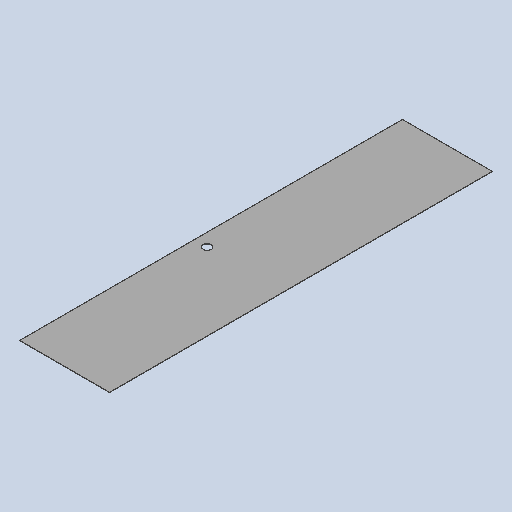
# Autodesk Inventor part: BSH 051 sheet in
Saved by Autodesk Inventor 2025 (Build 290162010, 162A)
## iProperties
Created: 2024-07-23
Part Number: BSH 051 sheet in
Material: 09g2s
Document SubType Name: Sheet Metal
Designer: admin
Mass: 40581.4 g
Surface Area: 34651.2 cm^2
Volume: 5169.6 cm^3
Density: 7.85 g/cm^3
Flat Pattern Width: 70 cm
Flat Pattern Length: 298 cm
Flat Pattern Area: 20860 cm^2
Sheet Metal Rule: AISI304 3mm Die 32
Sheet Metal Width: 700,000 mm
Sheet Metal Length: 2980,000 mm
Sheet Metal Area: 2086000,000 mm^2
Appearance: Default
Stock Number: БШК 051 лист внутренний
Author: admin
Autodesk Inventor part; units mm, degrees
ref_plane "YZ Plane" through (0, 0, 0) normal (1, 0, 0) x (0, 1, 0)
ref_plane "XZ Plane" through (0, 0, 0) normal (0, 1, 0) x (-1, 0, 0)
ref_plane "XY Plane" through (0, 0, 0) normal (0, 0, 1) x (1, 0, 0)
sketch "Sketch1" plane through (0, 0, 0) normal (0, 0, 1) x (1, 0, 0)
  line L0 (0, -1490) -> (700, -1490)
  line L1 (700, -1490) -> (700, 1490)
  line L2 (700, 1490) -> (0, 1490)
  line L3 (0, 1490) -> (0, -1490)
  point P0 (0, 0)
  point P1 (0, 0)
  dimension "d0" = 700
  dimension "d1" = 2980
  measures "d0" distance of L2.end L1.end
  measures "d1" distance of L1.end L0.end
extrude "Plate1" add sketch "Sketch1" along normal blind 3
sketch "Sketch6" plane through (0, 0, 3) normal (0, 0, 1) x (1, 0, 0)
  circle A0 centre (100, -130) radius 32.5
  line L0 (0, 1490) -> (700, 1490) projected
  line L1 (700, 1490) -> (700, -1490) projected
  line L2 (0, -1490) -> (0, 1490) projected
  point P0 (0, 0)
  point P1 (0, 0)
  dimension "d36" = 65
  dimension "d37" = 1620
  dimension "d41" = 100
  constraints: 1 centre point, 1 midpoint
  measures "d36" diameter of A0
  measures "d37" distance from line of L0 A0.centre
  measures "d41" horizontal distance of point (0, 0) A0.centre
extrude "Extrusion2" cut sketch "Sketch6" against normal up to surface (3 mm away)
equation "\"d2\" = Thickness"
equation "\"BendReliefWidth\" = Thickness"
equation "\"BendReliefDepth\" = 0.5 * Thickness"
equation "\"CornerReliefSize\" = 4 * Thickness"
equation "\"MinimumRemnant\" = 2 * Thickness"
equation "\"TransitionRadius\" = BendRadius"
equation "\"JacobiRadiusSize\" = BendRadius"
equation "\"GapSize\" = Thickness"
equation "\"Thickness\" = 3"
equation "\"BendRadius\" = 5"
body "Solid1"
